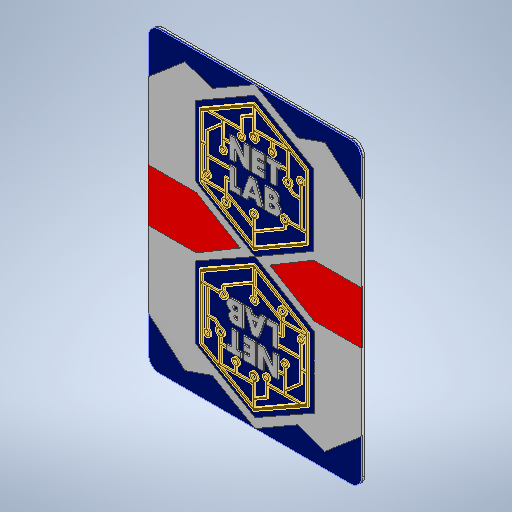
# Autodesk Inventor part: 3ofpython
Saved by Autodesk Inventor 2025 (Build 290162010, 162A)
## iProperties
Created: 2024-07-12
Part Number: 3ofpython
Material: Generic
Document SubType Name: Modeling
Designer: joshu
Density: 1 g/cm^3
Appearance: Default
Author: joshu
Autodesk Inventor part; units mm, degrees
(part 1 of 2)
ref_plane "YZ Plane" through (0, 0, 0) normal (1, 0, 0) x (0, 1, 0)
ref_plane "XZ Plane" through (0, 0, 0) normal (0, 1, 0) x (-1, 0, 0)
ref_plane "XY Plane" through (0, 0, 0) normal (0, 0, 1) x (1, 0, 0)
sketch "Sketch1" plane through (0, 0, 0) normal (0, 0, 1) x (1, 0, 0)
  line L0 (0, 0) -> (63.5, 0)
  line L1 (63.5, 0) -> (63.5, 88.9)
  line L2 (63.5, 88.9) -> (0, 88.9)
  line L3 (0, 88.9) -> (0, 0)
  line L4 (31.75, 44.45) -> (49.3079, 54.587)
  line L5 (49.3079, 54.587) -> (49.3079, 75.7826)
  line L6 (49.3079, 75.7826) -> (31.6801, 86.0828)
  line L7 (31.6801, 86.0828) -> (13.967, 75.8563)
  line L8 (13.967, 75.8563) -> (13.967, 55.04)
  line L9 (13.967, 55.04) -> (31.75, 44.45)
  line L10 (15.5263, 74.956) -> (31.6754, 84.2796)
  line L11 (31.6754, 84.2796) -> (47.7487, 74.8877)
  line L12 (47.7487, 74.8877) -> (47.7487, 55.4872)
  line L13 (47.7487, 55.4872) -> (31.7622, 46.2575)
  line L14 (31.7622, 46.2575) -> (15.5263, 55.9263)
  line L15 (15.5263, 55.9263) -> (15.5263, 74.956)
  line L16 (47.1273, 56.0392) -> (31.9379, 47.2671)
  line L17 (31.3664, 47.317) -> (16.2977, 56.192)
  line L18 (41.8086, 77.4972) -> (32.0418, 77.4972)
  line L19 (42.0908, 76.9257) -> (42.0908, 70.0939)
  line L20 (41.5193, 72.1376) -> (39.6994, 72.1376)
  line L21 (39.6994, 72.1376) -> (39.6994, 71.5661)
  line L22 (39.6994, 71.5661) -> (41.5193, 71.5661)
  arc A0 (31.465, 76.5861) -> (32.0365, 76.5861) centre (31.7507, 75.3324) ccw
  arc A1 (36.8763, 75.3571) -> (37.4478, 75.3571) centre (37.162, 74.2504) ccw
  circle A2 centre (37.162, 74.2504) radius 0.4762
  circle A3 centre (31.7507, 75.3324) radius 0.6191
  line L23 (45.9318, 69.8545) -> (45.9318, 58.9507)
  line L24 (45.3603, 66.7769) -> (43.3841, 66.7769)
  line L25 (43.1915, 66.2054) -> (45.3603, 66.2054)
  circle A4 centre (41.805, 68.7917) radius 0.762
  line L26 (43.1915, 66.2054) -> (41.9826, 67.4703)
  line L27 (43.3841, 66.7769) -> (42.5287, 67.6719)
  arc A5 (45.9318, 69.8545) -> (45.3603, 69.8545) centre (45.646, 70.9598) ccw
  circle A6 centre (45.646, 70.9598) radius 0.5715
  line L28 (40.6132, 56.5528) -> (40.6132, 57.4113)
  circle A7 centre (40.899, 58.665) radius 0.7144
  line L29 (32.0418, 83.1688) -> (32.0418, 77.4972)
  line L30 (32.0365, 76.9257) -> (32.0365, 76.5861)
  line L31 (32.0365, 76.9257) -> (36.8763, 76.9257)
  line L32 (36.8763, 75.3571) -> (36.8763, 76.9257)
  line L33 (37.4478, 76.9257) -> (37.4478, 75.3571)
  line L34 (37.4478, 76.9257) -> (41.5193, 76.9257)
  line L35 (42.0908, 76.9257) -> (42.7928, 76.9257)
  line L36 (32.0365, 83.1719) -> (41.8086, 77.4972)
  line L37 (42.7928, 76.9257) -> (47.1273, 74.4086)
  line L38 (41.5193, 70.0939) -> (41.5193, 71.5661)
  line L39 (41.5193, 72.1376) -> (41.5193, 76.9257)
  arc A8 (41.5193, 70.0939) -> (41.9826, 67.4703) centre (41.805, 68.7917) ccw
  arc A9 (42.5287, 67.6719) -> (42.0908, 70.0939) centre (41.805, 68.7917) ccw
  line L40 (45.3603, 58.9507) -> (45.3603, 66.2054)
  line L41 (45.3603, 66.7769) -> (45.3603, 69.8545)
  line L42 (47.1273, 58.9507) -> (45.9318, 58.9507)
  line L43 (45.3603, 58.9507) -> (42.1527, 58.9507)
  line L44 (42.1475, 58.3804) -> (47.1273, 58.3804)
  line L45 (41.1819, 57.4161) -> (41.1819, 56.2658)
  arc A10 (42.1527, 58.9507) -> (40.6132, 57.4113) centre (40.899, 58.665) ccw
  arc A11 (41.1819, 57.4161) -> (42.1475, 58.3804) centre (40.899, 58.665) ccw
  line L46 (47.1273, 74.4086) -> (47.1273, 58.9507)
  line L47 (47.1273, 58.3804) -> (47.1273, 56.0392)
  line L48 (27.6974, 78.6822) -> (27.6974, 79.0777)
  line L49 (28.2689, 78.6822) -> (31.465, 80.528)
  line L50 (27.6974, 79.0777) -> (31.465, 81.2535)
  line L51 (31.465, 76.5861) -> (31.465, 80.528)
  line L52 (31.465, 81.2535) -> (31.465, 83.1596)
  line L53 (31.9379, 51.4601) -> (40.6132, 56.5528)
  line L54 (31.9379, 50.8392) -> (41.1819, 56.2658)
  line L55 (16.2977, 57.1448) -> (22.9994, 57.1448)
  line L56 (22.9994, 56.5733) -> (16.2977, 56.5733)
  line L57 (16.2977, 56.5733) -> (16.2977, 57.1448)
  line L58 (22.9994, 60.9472) -> (23.5709, 60.9472)
  line L59 (22.9994, 60.9472) -> (24.4329, 60.9472)
  line L60 (24.4329, 60.9472) -> (24.4329, 60.3757)
  line L61 (24.4329, 60.3757) -> (23.5709, 60.3757)
  line L62 (22.9994, 60.3757) -> (22.9994, 60.9472)
  line L63 (23.5709, 56.4373) -> (31.3664, 51.9861)
  line L64 (31.3664, 52.5972) -> (23.5709, 57.0484)
  arc A12 (31.9379, 54.3552) -> (31.3664, 54.3552) centre (31.6521, 55.5111) ccw
  circle A13 centre (31.6521, 55.5111) radius 0.6191
  arc A14 (22.9994, 55.5805) -> (23.5709, 55.5805) centre (23.2852, 54.3309) ccw
  circle A15 centre (23.2852, 54.3309) radius 0.7144
  line L65 (23.5709, 60.3757) -> (23.5709, 57.0484)
  line L66 (23.5709, 56.4373) -> (23.5709, 55.5805)
  line L67 (22.9994, 55.5805) -> (22.9994, 56.5733)
  line L68 (22.9994, 57.1448) -> (22.9994, 60.9472)
  line L69 (31.3664, 54.3552) -> (31.3664, 52.5972)
  line L70 (31.3664, 51.9861) -> (31.3664, 47.317)
  line L71 (31.9379, 47.2671) -> (31.9379, 50.8392)
  line L72 (31.9379, 51.4601) -> (31.9379, 54.3552)
  arc A16 (27.6974, 74.6924) -> (28.2689, 74.6924) centre (27.9831, 73.6844) ccw
  circle A17 centre (27.9831, 73.6844) radius 0.4763
  line L73 (18.5492, 75.7007) -> (27.6974, 75.7007)
  line L74 (22.769, 70.6818) -> (24.4329, 70.6818)
  line L75 (24.4329, 70.6818) -> (24.4329, 70.1103)
  line L76 (24.4329, 70.1103) -> (22.769, 70.1103)
  line L77 (22.769, 70.1103) -> (22.769, 70.2009)
  line L78 (16.2977, 66.7769) -> (17.4065, 66.7769)
  line L79 (17.978, 66.7769) -> (17.978, 66.2054)
  line L80 (17.4065, 66.2054) -> (16.2977, 66.2054)
  line L81 (17.978, 63.9706) -> (24.4329, 63.9706)
  line L82 (24.4329, 63.9706) -> (24.4329, 63.3991)
  line L83 (24.4329, 63.3991) -> (17.978, 63.3991)
  line L84 (17.4065, 66.7769) -> (17.4065, 70.2549)
  line L85 (17.978, 70.0307) -> (17.978, 66.7769)
  line L86 (17.4065, 70.2549) -> (22.1975, 74.4365)
  line L87 (17.978, 70.0307) -> (22.1975, 73.7135)
  arc A18 (22.1975, 68.5281) -> (22.769, 68.5281) centre (22.4833, 67.4703) ccw
  circle A19 centre (22.4833, 67.4703) radius 0.5239
  line L88 (16.2977, 74.4004) -> (17.5596, 75.1292)
  line L89 (18.5492, 75.7007) -> (31.465, 83.1596)
  line L90 (27.6974, 75.1292) -> (22.769, 75.1292)
  line L91 (22.1975, 75.1292) -> (17.5596, 75.1292)
  line L92 (22.1975, 74.4365) -> (22.1975, 75.1292)
  line L93 (28.2689, 74.6924) -> (28.2689, 78.6822)
  line L94 (22.769, 75.1292) -> (22.769, 70.6818)
  line L95 (22.769, 70.1103) -> (22.769, 68.5281)
  line L96 (22.1975, 67.8875) -> (22.1975, 67.9094)
  line L97 (22.1975, 68.5281) -> (22.1975, 73.7135)
  line L98 (16.2977, 56.192) -> (16.2977, 66.2054)
  line L99 (16.2977, 66.7769) -> (16.2977, 74.4004)
  line L100 (17.978, 63.9706) -> (17.978, 66.2054)
  line L101 (27.6974, 78.6822) -> (27.6974, 75.7007)
  line L102 (27.6974, 75.1292) -> (27.6974, 74.6924)
  line L103 (24.4329, 66.1976) -> (26.1474, 66.1976)
  line L104 (26.1474, 66.1976) -> (26.1474, 69.7075)
  line L105 (26.1474, 72.4542) -> (24.4329, 72.4542)
  line L106 (24.4329, 72.4542) -> (24.4329, 66.1976)
  line L107 (28.7777, 72.4542) -> (30.4922, 72.4542)
  line L108 (30.4922, 72.4542) -> (30.4922, 66.1976)
  line L109 (30.4922, 66.1976) -> (28.7777, 66.1976)
  line L110 (28.7777, 68.9443) -> (28.7777, 72.4542)
  line L111 (28.7777, 66.1976) -> (26.1474, 69.7075)
  line L112 (26.1474, 72.4542) -> (28.7777, 68.9443)
  line L113 (31.2537, 72.4542) -> (32.9682, 72.4542)
  line L114 (32.9682, 66.1976) -> (31.2537, 66.1976)
  line L115 (31.2537, 66.1976) -> (31.2537, 72.4542)
  line L116 (31.2537, 72.4542) -> (34.8385, 72.4542)
  line L117 (34.8385, 72.4542) -> (34.8385, 70.7397)
  line L118 (34.8385, 70.7397) -> (32.9682, 70.7397)
  line L119 (31.2537, 70.7397) -> (31.2537, 72.4542)
  line L120 (32.9682, 70.0633) -> (34.8385, 70.0633)
  line L121 (34.8385, 70.0633) -> (34.8385, 68.5393)
  line L122 (34.8385, 68.5393) -> (32.9682, 68.5393)
  line L123 (31.2537, 68.5393) -> (31.2537, 70.0633)
  line L124 (31.2537, 66.1976) -> (34.8385, 66.1976)
  line L125 (34.8385, 66.1976) -> (34.8385, 67.9121)
  line L126 (34.8385, 67.9121) -> (32.9682, 67.9121)
  line L127 (31.2537, 67.9121) -> (31.2537, 66.1976)
  line L128 (32.9682, 70.7397) -> (32.9682, 70.0633)
  line L129 (32.9682, 68.5393) -> (32.9682, 67.9121)
  line L130 (39.6994, 72.4422) -> (35.4849, 72.4422)
  line L131 (35.4849, 72.4422) -> (35.4849, 70.9182)
  line L132 (39.6994, 70.9182) -> (39.6994, 72.4422)
  line L133 (38.4466, 70.9182) -> (38.4466, 66.1976)
  line L134 (38.4466, 66.1976) -> (36.7321, 66.1976)
  line L135 (36.7321, 66.1976) -> (36.7321, 70.9182)
  line L136 (36.7321, 70.9182) -> (36.8763, 70.9182)
  line L137 (35.4849, 70.9182) -> (36.7321, 70.9182)
  line L138 (38.4466, 70.9182) -> (39.6994, 70.9182)
  line L139 (24.4329, 64.6461) -> (26.1474, 64.6461)
  line L140 (26.1474, 64.6461) -> (26.1474, 59.9044)
  line L141 (26.1474, 58.3804) -> (24.4329, 58.3804)
  line L142 (24.4329, 58.3804) -> (24.4329, 64.6461)
  line L143 (24.4329, 58.3804) -> (27.8234, 58.3804)
  line L144 (27.8234, 58.3804) -> (27.8234, 59.9044)
  line L145 (27.8234, 59.9044) -> (26.1474, 59.9044)
  line L146 (24.4329, 59.9044) -> (24.4329, 58.3804)
  line L147 (28.1466, 58.3804) -> (29.8611, 58.3804)
  line L148 (29.8611, 58.3804) -> (30.3254, 59.5144)
  line L149 (30.3254, 59.5144) -> (32.2304, 59.5144)
  line L150 (30.3254, 64.6461) -> (32.2304, 64.6461)
  line L151 (28.1466, 58.3804) -> (30.3254, 64.6461)
  line L152 (32.728, 58.3804) -> (34.4425, 58.3804)
  line L153 (32.728, 58.3804) -> (32.2304, 59.5144)
  line L154 (34.4425, 58.3804) -> (32.2304, 64.6461)
  line L155 (30.6203, 60.8236) -> (31.9379, 60.8236)
  line L156 (31.9379, 60.8236) -> (31.2779, 62.4085)
  line L157 (31.2779, 62.4085) -> (30.6203, 60.8236)
  line L158 (34.9216, 58.3804) -> (34.9216, 64.6461)
  line L159 (34.9216, 64.6461) -> (37.8691, 64.6461)
  line L160 (34.9216, 58.3804) -> (37.8691, 58.3804)
  line L161 (36.5599, 59.8143) -> (36.5599, 60.939)
  line L162 (36.5599, 62.1736) -> (36.5599, 63.1944)
  line L163 (36.5599, 63.1944) -> (37.2133, 63.1944)
  line L164 (36.5599, 62.1736) -> (37.2133, 62.1736)
  arc A20 (37.2133, 62.1736) -> (37.2133, 63.1944) centre (37.055, 62.684) ccw
  line L165 (36.5599, 60.939) -> (37.4519, 60.939)
  line L166 (36.5599, 59.8143) -> (37.4396, 59.8143)
  arc A21 (37.4396, 59.8143) -> (37.4519, 60.939) centre (37.3959, 60.3772) ccw
  arc A22 (38.5631, 61.7817) -> (37.8691, 64.6461) centre (37.5266, 63.0469) ccw
  arc A23 (37.8691, 58.3804) -> (38.5631, 61.7817) centre (37.9604, 60.1332) ccw
  arc A24 (17.4065, 59.8724) -> (17.978, 59.8724) centre (17.6923, 58.815) ccw
  circle A25 centre (17.6923, 58.815) radius 0.5239
  line L167 (17.4065, 66.2054) -> (17.4065, 59.8724)
  line L168 (17.978, 59.8724) -> (17.978, 63.3991)
  line L169 (32.0418, 83.1688) -> (41.8086, 77.4972)
  line L170 (32.0418, 77.4972) -> (41.8086, 77.4972)
  line L171 (32.0418, 77.4972) -> (32.0418, 83.1688)
  line L172 (0, 44.45) -> (63.5, 44.45) construction
  line L173 (31.75, 88.9) -> (31.75, 0) construction
  line L174 (0, 52.2573) -> (14.2102, 52.2573)
  line L175 (14.2102, 52.2573) -> (27.3204, 44.45)
  line L176 (0, 36.6427) -> (14.2102, 36.6427)
  line L177 (14.2102, 36.6427) -> (27.3204, 44.45)
  line L178 (63.5, 52.2573) -> (49.2898, 52.2573)
  line L179 (49.2898, 52.2573) -> (36.1796, 44.45)
  line L180 (49.2898, 36.6427) -> (36.1796, 44.45)
  line L181 (63.5, 36.6427) -> (49.2898, 36.6427)
  line L182 (0, 75.0796) -> (10.8905, 84.3747)
  line L183 (10.8905, 84.3747) -> (18.9583, 81.5148)
  line L184 (18.9583, 81.5148) -> (31.75, 88.9)
  line L185 (63.5, 75.0796) -> (52.6095, 84.3747)
  line L186 (52.6095, 84.3747) -> (44.5417, 81.5148)
  line L187 (44.5417, 81.5148) -> (31.75, 88.9)
  line L188 (46.0393, 22.6946) -> (47.1481, 22.6946)
  line L189 (45.4678, 22.1231) -> (45.4678, 22.6946)
  line L190 (45.4678, 24.9294) -> (45.4678, 22.6946)
  line L191 (47.1481, 22.1231) -> (46.0393, 22.1231)
  line L192 (47.1481, 32.3267) -> (47.1481, 31.7552)
  line L193 (47.1481, 32.708) -> (47.1481, 22.6946)
  line L194 (47.1481, 31.7552) -> (40.4464, 31.7552)
  line L195 (40.4464, 32.3267) -> (47.1481, 32.3267)
  line L196 (45.4678, 29.0276) -> (45.4678, 25.5009)
  line L197 (46.0393, 22.6946) -> (46.0393, 29.0276)
  circle A26 centre (45.7535, 30.085) radius 0.5239
  arc A27 (46.0393, 29.0276) -> (45.4678, 29.0276) centre (45.7535, 30.085) ccw
  line L198 (20.6531, 11.9743) -> (16.3185, 14.4914)
  line L199 (21.355, 11.9743) -> (20.6531, 11.9743)
  line L200 (21.9265, 16.7624) -> (21.9265, 11.9743)
  line L201 (21.355, 11.9743) -> (21.355, 18.8061)
  line L202 (21.9265, 16.7624) -> (23.7464, 16.7624)
  line L203 (23.7464, 17.3339) -> (21.9265, 17.3339)
  line L204 (25.998, 11.9743) -> (21.9265, 11.9743)
  line L205 (26.5695, 13.5429) -> (26.5695, 11.9743)
  circle A28 centre (21.6408, 20.1083) radius 0.762
  circle A29 centre (26.2838, 14.6496) radius 0.4762
  arc A30 (26.5695, 13.5429) -> (25.998, 13.5429) centre (26.2838, 14.6496) ccw
  line L206 (31.4093, 11.9743) -> (26.5695, 11.9743)
  arc A31 (31.9808, 12.3139) -> (31.4093, 12.3139) centre (31.6951, 13.5676) ccw
  line L207 (25.998, 11.9743) -> (25.998, 13.5429)
  line L208 (45.4678, 24.9294) -> (39.013, 24.9294)
  line L209 (39.013, 25.5009) -> (45.4678, 25.5009)
  line L210 (39.013, 24.9294) -> (39.013, 25.5009)
  circle A32 centre (40.1606, 34.5691) radius 0.7144
  arc A33 (40.4464, 33.3195) -> (39.8749, 33.3195) centre (40.1606, 34.5691) ccw
  line L211 (39.8749, 32.4627) -> (39.8749, 33.3195)
  line L212 (40.4464, 33.3195) -> (40.4464, 32.3267)
  line L213 (39.013, 27.9528) -> (39.013, 28.5243)
  line L214 (39.8749, 28.5243) -> (39.8749, 31.8516)
  line L215 (39.013, 28.5243) -> (39.8749, 28.5243)
  line L216 (40.4464, 31.7552) -> (40.4464, 27.9528)
  line L217 (40.4464, 28.5243) -> (40.4464, 27.9528)
  line L218 (40.4464, 27.9528) -> (39.8749, 27.9528)
  line L219 (40.4464, 27.9528) -> (39.013, 27.9528)
  line L220 (33.5847, 30.5196) -> (33.1204, 29.3856)
  line L221 (35.6224, 28.9956) -> (37.2985, 28.9956)
  line L222 (35.2992, 30.5196) -> (33.5847, 30.5196)
  line L223 (39.013, 28.9956) -> (39.013, 30.5196)
  line L224 (35.2992, 30.5196) -> (33.1204, 24.2539)
  line L225 (46.0393, 18.6451) -> (41.2483, 14.4635)
  line L226 (45.4678, 18.8693) -> (41.2483, 15.1865)
  line L227 (40.6768, 18.7897) -> (40.6768, 20.3719)
  line L228 (41.2483, 21.0125) -> (41.2483, 20.9906)
  line L229 (41.2483, 20.3719) -> (41.2483, 15.1865)
  line L230 (40.6768, 13.7708) -> (40.6768, 18.2182)
  line L231 (41.2483, 14.4635) -> (41.2483, 13.7708)
  line L232 (41.2483, 13.7708) -> (45.8862, 13.7708)
  line L233 (47.1481, 22.1231) -> (47.1481, 14.4996)
  line L234 (47.1481, 14.4996) -> (45.8862, 13.7708)
  circle A34 centre (40.9626, 21.4297) radius 0.5239
  line L235 (32.8255, 28.0764) -> (31.5079, 28.0764)
  line L236 (32.1679, 26.4915) -> (32.8255, 28.0764)
  line L237 (31.5079, 28.0764) -> (32.1679, 26.4915)
  line L238 (33.1204, 29.3856) -> (31.2154, 29.3856)
  line L239 (35.6224, 30.5196) -> (35.6224, 28.9956)
  line L240 (37.2985, 24.2539) -> (37.2985, 28.9956)
  line L241 (37.2985, 30.5196) -> (39.013, 30.5196)
  line L242 (39.013, 30.5196) -> (39.013, 24.2539)
  line L243 (39.013, 30.5196) -> (35.6224, 30.5196)
  line L244 (39.013, 24.2539) -> (37.2985, 24.2539)
  line L245 (33.1204, 24.2539) -> (31.2154, 24.2539)
  line L246 (30.7178, 30.5196) -> (31.2154, 29.3856)
  line L247 (37.2985, 16.4458) -> (39.013, 16.4458)
  line L248 (40.6768, 18.2182) -> (39.013, 18.2182)
  line L249 (39.013, 18.7897) -> (40.6768, 18.7897)
  line L250 (40.6768, 18.7897) -> (40.6768, 18.6991)
  line L251 (39.013, 18.2182) -> (39.013, 18.7897)
  line L252 (46.0393, 22.1231) -> (46.0393, 18.6451)
  line L253 (45.4678, 18.8693) -> (45.4678, 22.1231)
  arc A35 (41.2483, 20.3719) -> (40.6768, 20.3719) centre (40.9626, 21.4297) ccw
  line L254 (39.013, 16.4458) -> (39.013, 22.7024)
  line L255 (39.013, 22.7024) -> (37.2985, 22.7024)
  line L256 (32.9536, 22.7024) -> (34.6681, 22.7024)
  line L257 (30.4777, 22.7024) -> (32.1922, 22.7024)
  line L258 (30.4777, 18.8367) -> (28.6073, 18.8367)
  line L259 (32.1922, 22.7024) -> (28.6073, 22.7024)
  line L260 (28.6073, 22.7024) -> (28.6073, 20.9879)
  line L261 (28.6073, 20.9879) -> (30.4777, 20.9879)
  line L262 (32.1922, 20.9879) -> (32.1922, 22.7024)
  line L263 (30.4777, 20.3607) -> (30.4777, 20.9879)
  line L264 (28.6073, 20.3607) -> (30.4777, 20.3607)
  line L265 (28.6073, 18.8367) -> (28.6073, 20.3607)
  line L266 (32.1922, 20.3607) -> (32.1922, 18.8367)
  line L267 (30.4777, 18.1603) -> (30.4777, 18.8367)
  line L268 (26.8859, 25.7056) -> (26.2325, 25.7056)
  line L269 (26.8859, 29.0857) -> (26.0062, 29.0857)
  line L270 (26.8859, 27.961) -> (25.9939, 27.961)
  line L271 (28.5242, 30.5196) -> (25.5767, 30.5196)
  line L272 (32.0794, 36.9139) -> (32.0794, 41.583)
  line L273 (31.5079, 41.6329) -> (31.5079, 38.0608)
  line L274 (26.8859, 26.7264) -> (26.8859, 25.7056)
  line L275 (28.5242, 24.2539) -> (25.5767, 24.2539)
  line L276 (29.0033, 30.5196) -> (31.2154, 24.2539)
  line L277 (30.7178, 30.5196) -> (29.0033, 30.5196)
  line L278 (26.8859, 26.7264) -> (26.2325, 26.7264)
  line L279 (28.5242, 30.5196) -> (28.5242, 24.2539)
  arc A36 (26.2325, 26.7264) -> (26.2325, 25.7056) centre (26.3908, 26.216) ccw
  line L280 (26.8859, 29.0857) -> (26.8859, 27.961)
  arc A37 (26.0062, 29.0857) -> (25.9939, 27.961) centre (26.0499, 28.5228) ccw
  arc A38 (24.8827, 27.1183) -> (25.5767, 24.2539) centre (25.9192, 25.8531) ccw
  arc A39 (25.5767, 30.5196) -> (24.8827, 27.1183) centre (25.4854, 28.7668) ccw
  line L281 (23.7464, 16.7624) -> (23.7464, 17.3339)
  line L282 (24.9992, 22.7024) -> (26.7137, 22.7024)
  line L283 (27.961, 17.9818) -> (26.7137, 17.9818)
  line L284 (26.7137, 22.7024) -> (26.7137, 17.9818)
  line L285 (26.7137, 17.9818) -> (26.5695, 17.9818)
  line L286 (24.9992, 17.9818) -> (24.9992, 22.7024)
  line L287 (24.9992, 17.9818) -> (23.7464, 17.9818)
  line L288 (27.961, 16.4578) -> (27.961, 17.9818)
  line L289 (23.7464, 16.4578) -> (27.961, 16.4578)
  line L290 (23.7464, 17.9818) -> (23.7464, 16.4578)
  line L291 (31.75, 44.45) -> (14.1379, 34.5158)
  line L292 (15.6972, 33.6051) -> (31.7276, 42.6471)
  line L293 (16.3185, 32.8608) -> (31.5079, 41.6329)
  line L294 (31.5079, 37.4399) -> (22.8326, 32.3472)
  line L295 (31.5079, 38.0608) -> (22.2639, 32.6342)
  line L296 (31.5079, 37.4399) -> (31.5079, 34.5448)
  line L297 (35.7484, 10.2178) -> (35.7484, 9.8223)
  line L298 (35.1769, 10.2178) -> (31.9808, 8.372)
  line L299 (35.7484, 9.8223) -> (31.9808, 7.6465)
  line L300 (31.9808, 12.3139) -> (31.9808, 8.372)
  line L301 (31.9808, 7.6465) -> (31.9808, 5.7404)
  circle A40 centre (35.4627, 15.2156) radius 0.4763
  arc A41 (35.7484, 14.2076) -> (35.1769, 14.2076) centre (35.4627, 15.2156) ccw
  line L302 (35.7484, 13.7708) -> (35.7484, 14.2076)
  line L303 (35.7484, 13.7708) -> (40.6768, 13.7708)
  line L304 (44.8966, 13.1993) -> (35.7484, 13.1993)
  line L305 (35.1769, 14.2076) -> (35.1769, 10.2178)
  line L306 (35.7484, 10.2178) -> (35.7484, 13.1993)
  line L307 (44.8966, 13.1993) -> (31.9808, 5.7404)
  line L308 (31.4093, 11.9743) -> (31.4093, 12.3139)
  line L309 (47.9195, 13.7706) -> (31.7623, 4.657)
  circle A42 centre (31.6951, 13.5676) radius 0.6191
  line L310 (31.7499, 2.8598) -> (49.4788, 12.8599)
  line L311 (47.9195, 32.9751) -> (47.9195, 13.7706)
  line L312 (49.4788, 12.8599) -> (49.4788, 33.86)
  circle A43 centre (31.7937, 33.3889) radius 0.6191
  line L313 (32.0794, 41.583) -> (47.1481, 32.708)
  line L314 (49.4788, 33.86) -> (31.75, 44.45)
  line L315 (31.7276, 42.6471) -> (47.9195, 32.9751)
  line L316 (32.0794, 36.3028) -> (39.8749, 31.8516)
  line L317 (39.8749, 32.4627) -> (32.0794, 36.9139)
  line L318 (32.0794, 34.5448) -> (32.0794, 36.3028)
  arc A44 (31.5079, 34.5448) -> (32.0794, 34.5448) centre (31.7937, 33.3889) ccw
  circle A45 centre (17.7998, 17.9402) radius 0.5715
  line L319 (18.0855, 22.1231) -> (20.0617, 22.1231)
  line L320 (20.2543, 22.6946) -> (18.0855, 22.6946)
  line L321 (22.8326, 32.3472) -> (22.8326, 31.4887)
  circle A46 centre (22.5468, 30.235) radius 0.7144
  line L322 (21.2984, 30.5196) -> (16.3185, 30.5196)
  line L323 (22.2639, 31.4839) -> (22.2639, 32.6342)
  arc A47 (21.2931, 29.9493) -> (22.8326, 31.4887) centre (22.5468, 30.235) ccw
  arc A48 (22.2639, 31.4839) -> (21.2984, 30.5196) centre (22.5468, 30.235) ccw
  line L324 (16.3185, 30.5196) -> (16.3185, 32.8608)
  line L325 (14.1379, 34.5158) -> (14.1379, 13.1174)
  line L326 (15.6972, 14.0137) -> (15.6972, 33.6051)
  line L327 (17.514, 19.0455) -> (17.514, 29.9493)
  line L328 (20.2543, 22.6946) -> (21.4633, 21.4297)
  line L329 (20.0617, 22.1231) -> (20.9171, 21.2281)
  arc A49 (17.514, 19.0455) -> (18.0855, 19.0455) centre (17.7998, 17.9402) ccw
  line L330 (21.9265, 18.8061) -> (21.9265, 17.3339)
  arc A50 (20.9171, 21.2281) -> (21.355, 18.8061) centre (21.6408, 20.1083) ccw
  line L331 (18.0855, 22.1231) -> (18.0855, 19.0455)
  line L332 (16.3185, 14.4914) -> (16.3185, 29.9493)
  line L333 (16.3185, 29.9493) -> (17.514, 29.9493)
  line L334 (18.0855, 29.9493) -> (18.0855, 22.6946)
  line L335 (18.0855, 29.9493) -> (21.2931, 29.9493)
  arc A51 (21.9265, 18.8061) -> (21.4633, 21.4297) centre (21.6408, 20.1083) ccw
  line L336 (14.1379, 13.1174) -> (31.7499, 2.8598)
  line L337 (31.7623, 4.657) -> (15.6972, 14.0137)
  line L338 (21.6372, 11.4028) -> (31.404, 11.4028)
  line L339 (31.404, 11.4028) -> (31.404, 5.7312)
  line L340 (31.404, 5.7312) -> (21.6372, 11.4028)
  line L341 (37.2985, 22.7024) -> (37.2985, 19.1925)
  line L342 (34.6681, 16.4458) -> (32.9536, 16.4458)
  line L343 (32.9536, 16.4458) -> (32.9536, 22.7024)
  line L344 (34.6681, 22.7024) -> (37.2985, 19.1925)
  line L345 (28.6073, 18.1603) -> (30.4777, 18.1603)
  line L346 (32.1922, 16.4458) -> (28.6073, 16.4458)
  line L347 (28.6073, 16.4458) -> (28.6073, 18.1603)
  line L348 (32.1922, 22.7024) -> (32.1922, 16.4458)
  line L349 (32.1922, 16.4458) -> (30.4777, 16.4458)
  line L350 (34.6681, 19.9557) -> (34.6681, 16.4458)
  line L351 (37.2985, 16.4458) -> (34.6681, 19.9557)
  line L352 (32.1922, 18.1603) -> (32.1922, 16.4458)
  line L353 (0, 13.8204) -> (10.8905, 4.5253)
  line L354 (10.8905, 4.5253) -> (18.9583, 7.3852)
  line L355 (18.9583, 7.3852) -> (31.75, 0)
  line L356 (63.5, 13.8204) -> (52.6095, 4.5253)
  line L357 (52.6095, 4.5253) -> (44.5417, 7.3852)
  line L358 (44.5417, 7.3852) -> (31.75, 0)
  point P0 (31.9379, 47.317)
  point P1 (31.7229, 65.2666)
  point P2 (31.7229, 23.6334)
  point P3 (31.7229, 23.6334)
  point P4 (31.9379, 5.6837)
  point P5 (63.5, 75.0796)
  dimension "d0" = 63.5
  dimension "d1" = 88.9
  dimension "d43" = 44.45
  dimension "d99" = 120
  constraints: 718 end point, 170 parallel, 64 point on circle, 50 centre point, 42 perpendicular, 36 horizontal, 21 point on line, 20 coincident, 19 symmetric about line, 7 collinear, 5 midpoint, 4 vertical, 17 other
  measures "d0" distance of L2.end L1.end
  measures "d1" distance of L1.end L0.end
  measures "d43" distance between parallel lines of L172 L2
  measures "d99" angle of L357 L356
extrude "Extrusion1" add sketch "Sketch1" along normal blind 0.4 contours L3 L353 L354 L355 L0 | L358 L357 L356 L1 L0 | L3 L2 L184 L183 L182 | L185 L186 L187 L2 L1 | L9 L8 L7 L6 L5 L4 | L314 L312 L310 L336 L325 L291 | L10 L11 L12 L13 L14 L15 | L16 L71 L54 L45 A11 L44 L47 | L17 L98 L56 L67 A14 L66 L63 L70 | L18 L29 L36 | L35 L37 L46 L42 L23 A5 L41 L24 L27 A9 L19 | L20 L132 L130 L131 L137 L135 L134 L133 L138 L22 L38 A8 L26 L25 L40 L43 A10 L28 L53 L72 A12 L69 L64 L65 L61 L142 L141 L143 L144 L145 L140 L139 L81 L100 L79 L85 L87 L97 A18 L95 L76 L106 L103 L104 L111 L109 L108 L107 L110 L112 L105 L74 L94 L90 L102 A16 L93 L49 L51 A0 L30 L31 L32 A1 L33 L34 L39 | L21 L132 L138 L133 L134 L135 L137 L131 L130 | L106 L105 L112 L110 L107 L108 L109 L111 L104 L103 L75 | L60 L142 L82 L139 L140 L145 L144 L143 L141 | L59 L58 L62 L68 L55 L98 L80 L167 A24 L168 L83 L142 | A2 | A3 | A4 | A6 | A7 | L101 L73 L89 L52 L50 L48 | A13 | A15 | A17 | L99 L88 L91 L92 L86 L84 L78 | A19 | L113 L116 L117 L118 L128 L120 L121 L122 L129 L126 L125 L124 L114 L115 | L151 L150 L154 L152 L153 L149 L148 L147 | L157 L156 L155 | L158 L159 A22 A23 L160 | L161 L165 A21 L166 | L162 L163 A20 L164 | A25 | L197 A27 L196 L209 L242 L219 L218 L216 L194 L193 L188 | L210 L242 L244 L240 L221 L239 L243 L241 L223 L213 | L208 L190 L189 L253 L226 L229 A35 L227 L249 L254 L255 L341 L344 L256 L343 L342 L350 L351 L247 L248 L230 L303 L302 A41 L305 L298 L300 A31 L308 L206 L205 A30 L207 L204 L200 L202 L290 L289 L288 L283 L284 L282 L286 L287 L203 L330 A51 L328 L320 L334 L335 A47 L321 L294 L296 A44 L318 L316 L214 L215 L242 L223 L241 L243 L239 L221 L240 L244 | L251 L254 L247 L351 L350 L342 L343 L256 L344 L341 L255 | L290 L287 L286 L282 L284 L283 L288 L289 L281 | L233 L234 L232 L231 L225 L252 L191 | L193 L195 L212 A33 L211 L317 L272 L313 | A26 | L198 L332 L333 L327 A49 L331 L319 L329 A50 L201 L199 | A28 | A29 | A32 | L222 L224 L245 L276 L277 L246 L238 L220 | A34 | L236 L237 L235 | L257 L262 L348 L266 L346 L347 L345 L267 L258 L265 L264 L263 L261 L260 L259 | L268 A36 L278 L274 | L280 L270 A37 L269 | L279 L275 A38 A39 L271 | L273 L295 L323 A48 L322 L324 L293 | L292 L315 L311 L309 L337 L326 | L306 L304 L307 L301 L299 L297 | A40 | A42 | A43 | A45 | A46 | L338 L339 L340
extrude "Extrusion12" add sketch "Sketch1" along normal blind 0.4 separate body contours L3 L174 L175 L177 L176 | L181 L180 L179 L178 L1
extrude "Extrusion13" add sketch "Sketch1" along normal blind 0.4 separate body contours L355 L354 L353 L3 L176 L177 L175 L174 L182 L183 L184 L187 L186 L185 L1 L178 L179 L180 L181 L356 L357 L358
extrude "Extrusion14" add sketch "Sketch1" against normal blind 0.4 contours L21 L132 L138 L133 L134 L135 L137 L131 L130 | L106 L105 L112 L110 L107 L108 L109 L111 L104 L103 L75 | L60 L142 L82 L139 L140 L145 L144 L143 L141 | L113 L116 L117 L118 L128 L120 L121 L122 L129 L126 L125 L124 L114 L115 | L151 L150 L154 L152 L153 L149 L148 L147 | L158 L159 A22 A23 L160 | L210 L242 L244 L240 L221 L239 L243 L241 L223 L213 | L251 L254 L247 L351 L350 L342 L343 L256 L344 L341 L255 | L290 L287 L286 L282 L284 L283 L288 L289 L281 | L222 L224 L245 L276 L277 L246 L238 L220 | L257 L262 L348 L266 L346 L347 L345 L267 L258 L265 L264 L263 L261 L260 L259 | L279 L275 A38 A39 L271 bodies 3
extrude "Extrusion15" add sketch "Sketch1" against normal blind 0.4 separate body contours L10 L11 L12 L13 L14 L15 | L292 L315 L311 L309 L337 L326
pattern_linear "Rectangular Pattern1" count 2 spacing 0.8 along (0, 0, 1) of "Extrusion15" bodies 4
pattern_linear "Rectangular Pattern2" count 2 spacing 0.8 along (0, 0, 1) of "Extrusion14" bodies 3
extrude "Extrusion16" cut sketch "Sketch1" against normal blind 0.4 contours L9 L8 L7 L6 L5 L4 | L314 L312 L310 L336 L325 L291 | L10 L11 L12 L13 L14 L15 | L16 L71 L54 L45 A11 L44 L47 | L17 L98 L56 L67 A14 L66 L63 L70 | L18 L29 L36 | L35 L37 L46 L42 L23 A5 L41 L24 L27 A9 L19 | L20 L132 L130 L131 L137 L135 L134 L133 L138 L22 L38 A8 L26 L25 L40 L43 A10 L28 L53 L72 A12 L69 L64 L65 L61 L142 L141 L143 L144 L145 L140 L139 L81 L100 L79 L85 L87 L97 A18 L95 L76 L106 L103 L104 L111 L109 L108 L107 L110 L112 L105 L74 L94 L90 L102 A16 L93 L49 L51 A0 L30 L31 L32 A1 L33 L34 L39 | L21 L132 L138 L133 L134 L135 L137 L131 L130 | L106 L105 L112 L110 L107 L108 L109 L111 L104 L103 L75 | L60 L142 L82 L139 L140 L145 L144 L143 L141 | L59 L58 L62 L68 L55 L98 L80 L167 A24 L168 L83 L142 | A2 | A3 | A4 | A6 | A7 | L101 L73 L89 L52 L50 L48 | A13 | A15 | A17 | L99 L88 L91 L92 L86 L84 L78 | A19 | L113 L116 L117 L118 L128 L120 L121 L122 L129 L126 L125 L124 L114 L115 | L151 L150 L154 L152 L153 L149 L148 L147 | L157 L156 L155 | L158 L159 A22 A23 L160 | L161 L165 A21 L166 | L162 L163 A20 L164 | A25 | L197 A27 L196 L209 L242 L219 L218 L216 L194 L193 L188 | L210 L242 L244 L240 L221 L239 L243 L241 L223 L213 | L208 L190 L189 L253 L226 L229 A35 L227 L249 L254 L255 L341 L344 L256 L343 L342 L350 L351 L247 L248 L230 L303 L302 A41 L305 L298 L300 A31 L308 L206 L205 A30 L207 L204 L200 L202 L290 L289 L288 L283 L284 L282 L286 L287 L203 L330 A51 L328 L320 L334 L335 A47 L321 L294 L296 A44 L318 L316 L214 L215 L242 L223 L241 L243 L239 L221 L240 L244 | L251 L254 L247 L351 L350 L342 L343 L256 L344 L341 L255 | L290 L287 L286 L282 L284 L283 L288 L289 L281 | L233 L234 L232 L231 L225 L252 L191 | L193 L195 L212 A33 L211 L317 L272 L313 | A26 | L198 L332 L333 L327 A49 L331 L319 L329 A50 L201 L199 | A28 | A29 | A32 | L222 L224 L245 L276 L277 L246 L238 L220 | A34 | L236 L237 L235 | L257 L262 L348 L266 L346 L347 L345 L267 L258 L265 L264 L263 L261 L260 L259 | L268 A36 L278 L274 | L280 L270 A37 L269 | L279 L275 A38 A39 L271 | L273 L295 L323 A48 L322 L324 L293 | L292 L315 L311 L309 L337 L326 | L306 L304 L307 L301 L299 L297 | A40 | A42 | A43 | A45 | A46 | L338 L339 L340 bodies 3
extrude "Extrusion17" cut sketch "Sketch1" against normal blind 25.4 contours L9 L8 L7 L6 L5 L4 | L314 L312 L310 L336 L325 L291 | L10 L11 L12 L13 L14 L15 | L16 L71 L54 L45 A11 L44 L47 | L17 L98 L56 L67 A14 L66 L63 L70 | L18 L29 L36 | L35 L37 L46 L42 L23 A5 L41 L24 L27 A9 L19 | L20 L132 L130 L131 L137 L135 L134 L133 L138 L22 L38 A8 L26 L25 L40 L43 A10 L28 L53 L72 A12 L69 L64 L65 L61 L142 L141 L143 L144 L145 L140 L139 L81 L100 L79 L85 L87 L97 A18 L95 L76 L106 L103 L104 L111 L109 L108 L107 L110 L112 L105 L74 L94 L90 L102 A16 L93 L49 L51 A0 L30 L31 L32 A1 L33 L34 L39 | L21 L132 L138 L133 L134 L135 L137 L131 L130 | L106 L105 L112 L110 L107 L108 L109 L111 L104 L103 L75 | L60 L142 L82 L139 L140 L145 L144 L143 L141 | L59 L58 L62 L68 L55 L98 L80 L167 A24 L168 L83 L142 | A2 | A3 | A4 | A6 | A7 | L101 L73 L89 L52 L50 L48 | A13 | A15 | A17 | L99 L88 L91 L92 L86 L84 L78 | A19 | L113 L116 L117 L118 L128 L120 L121 L122 L129 L126 L125 L124 L114 L115 | L151 L150 L154 L152 L153 L149 L148 L147 | L157 L156 L155 | L158 L159 A22 A23 L160 | L161 L165 A21 L166 | L162 L163 A20 L164 | A25 | L197 A27 L196 L209 L242 L219 L218 L216 L194 L193 L188 | L210 L242 L244 L240 L221 L239 L243 L241 L223 L213 | L208 L190 L189 L253 L226 L229 A35 L227 L249 L254 L255 L341 L344 L256 L343 L342 L350 L351 L247 L248 L230 L303 L302 A41 L305 L298 L300 A31 L308 L206 L205 A30 L207 L204 L200 L202 L290 L289 L288 L283 L284 L282 L286 L287 L203 L330 A51 L328 L320 L334 L335 A47 L321 L294 L296 A44 L318 L316 L214 L215 L242 L223 L241 L243 L239 L221 L240 L244 | L251 L254 L247 L351 L350 L342 L343 L256 L344 L341 L255 | L290 L287 L286 L282 L284 L283 L288 L289 L281 | L233 L234 L232 L231 L225 L252 L191 | L193 L195 L212 A33 L211 L317 L272 L313 | A26 | L198 L332 L333 L327 A49 L331 L319 L329 A50 L201 L199 | A28 | A29 | A32 | L222 L224 L245 L276 L277 L246 L238 L220 | A34 | L236 L237 L235 | L257 L262 L348 L266 L346 L347 L345 L267 L258 L265 L264 L263 L261 L260 L259 | L268 A36 L278 L274 | L280 L270 A37 L269 | L279 L275 A38 A39 L271 | L273 L295 L323 A48 L322 L324 L293 | L292 L315 L311 L309 L337 L326 | L306 L304 L307 L301 L299 L297 | A40 | A42 | A43 | A45 | A46 | L338 L339 L340 bodies 4
sketch "Sketch14" plane through (0, 0, 0) normal (0, 0, -1) x (-1, 0, 0)
  line L0 (-63.5, 75.0796) -> (-63.5, 88.9) projected
  line L1 (0, 0) -> (-63.5, 0)
  line L2 (-63.5, 0) -> (-63.5, 88.9)
  line L3 (-63.5, 88.9) -> (0, 88.9)
  line L4 (0, 88.9) -> (0, 0)
  line L5 (-62.5, 1) -> (-1, 1)
  line L6 (-1, 1) -> (-1, 87.9)
  line L7 (-1, 87.9) -> (-62.5, 87.9)
  line L8 (-62.5, 87.9) -> (-62.5, 1)
  dimension "d90" = 1
  constraints: 16 end point, 4 parallel, 2 perpendicular, 1 horizontal, 3 other
  measures "d90" distance between parallel lines of L1 L5
extrude "Extrusion18" add sketch "Sketch14" along normal blind 0.2 separate body contours L8 L7 L6 L5
sketch "Sketch16" plane through (0, 0, 0) normal (0, 0, -1) x (-1, 0, 0)
  line L0 (-1, 1) -> (-1, 87.9) projected
  line L1 (-1, 87.9) -> (-62.5, 87.9) projected
  line L2 (-62.5, 87.9) -> (-62.5, 1) projected
  line L3 (-62.5, 1) -> (-1, 1) projected
  line L4 (0, 88.9) -> (0, 75.0796) projected
  line L5 (-31.75, 0) -> (-63.5, 0) projected
  line L6 (0, 88.9) -> (-63.5, 88.9)
  line L7 (-63.5, 88.9) -> (-63.5, 0)
  line L8 (-63.5, 0) -> (0, 0)
  line L9 (0, 0) -> (0, 88.9)
  constraints: 8 end point, 2 parallel, 1 horizontal, 1 perpendicular
extrude "Extrusion19" add sketch "Sketch16" along normal blind 0.2 bodies 3
sketch "Sketch17" plane through (0, 0, -0.2) normal (0, 0, -1) x (-1, 0, 0)
  line L0 (-63.5, 88.9) -> (-63.5, 0)
  line L1 (-63.5, 0) -> (0, 0)
  line L2 (0, 0) -> (0, 88.9)
  line L3 (0, 88.9) -> (-63.5, 88.9)
  line L4 (-62.5, 1) -> (-62.5, 87.9) construction
  line L5 (-62.5, 44.45) -> (-1, 44.45) construction
  line L6 (-1, 87.9) -> (-1, 1) construction
  line L7 (-57.9556, 87.392) -> (-49.5403, 87.392) construction
  line L8 (-49.5403, 87.392) -> (-49.5403, 73.7102) construction
  line L9 (-49.5403, 73.7102) -> (-57.9556, 73.7102) construction
  line L10 (-57.9556, 73.7102) -> (-57.9556, 87.392) construction
  line L11 (-5.5444, 1.508) -> (-13.9597, 1.508) construction
  line L12 (-13.9597, 1.508) -> (-13.9597, 15.8789) construction
  line L13 (-13.9597, 15.8789) -> (-5.5444, 15.8789) construction
  line L14 (-5.5444, 15.8789) -> (-5.5444, 1.508) construction
  line L15 (-62.5, 87.9) -> (-1, 87.9) projected
  line L16 (-1, 1) -> (-62.5, 1) projected
  line L17 (-15.9555, 100.6878) -> (-15.9555, 101.8081)
  arc A0 (-15.758, 102.5167) -> (-15.9555, 101.8081) centre (-14.5235, 101.7908) ccw
  arc A1 (-14.8139, 103.0351) -> (-15.758, 102.5167) centre (-14.7944, 101.8807) ccw
  line L18 (-14.8139, 103.0351) -> (-12.5434, 103.0404)
  arc A2 (-12.5434, 103.0404) -> (-11.3034, 104.2101) centre (-12.4298, 104.1621) ccw
  line L19 (-11.3034, 104.2101) -> (-11.308, 106.1909)
  arc A3 (-11.308, 106.1909) -> (-11.7101, 106.9805) centre (-12.2888, 106.1886) ccw
  arc A4 (-11.7101, 106.9805) -> (-12.7195, 107.3451) centre (-13.0065, 104.9711) ccw
  arc A5 (-12.7195, 107.3451) -> (-14.3215, 107.3451) centre (-13.5205, 101.117) ccw
  arc A6 (-14.3215, 107.3451) -> (-15.3501, 106.9805) centre (-14.123, 105.152) ccw
  arc A7 (-15.3501, 106.9805) -> (-15.6604, 106.4938) centre (-14.9717, 106.397) ccw
  line L20 (-15.6604, 106.4938) -> (-15.6604, 105.3776)
  line L21 (-15.6604, 105.3776) -> (-13.4817, 105.3776)
  line L22 (-13.4817, 105.3776) -> (-13.4817, 105.0592)
  line L23 (-13.4817, 105.0592) -> (-16.5554, 105.0592)
  arc A8 (-16.5554, 105.0592) -> (-17.8802, 103.9116) centre (-16.4912, 103.6466) ccw
  arc A9 (-17.8802, 103.9116) -> (-17.7338, 101.4545) centre (-14.109, 102.9033) ccw
  arc A10 (-17.7338, 101.4545) -> (-16.815, 100.6878) centre (-16.5647, 101.9218) ccw
  line L24 (-16.815, 100.6878) -> (-15.9555, 100.6878)
  line L25 (-10.9984, 105.1392) -> (-10.9984, 104.019)
  arc A11 (-11.1959, 103.3104) -> (-10.9984, 104.019) centre (-12.4304, 104.0362) ccw
  arc A12 (-12.14, 102.792) -> (-11.1959, 103.3104) centre (-12.1595, 103.9464) ccw
  line L26 (-12.14, 102.792) -> (-14.4105, 102.7867)
  arc A13 (-14.4105, 102.7867) -> (-15.6506, 101.6169) centre (-14.5241, 101.6649) ccw
  line L27 (-15.6506, 101.6169) -> (-15.6459, 99.6361)
  arc A14 (-15.6459, 99.6361) -> (-15.2438, 98.8466) centre (-14.6652, 99.6384) ccw
  arc A15 (-15.2438, 98.8466) -> (-14.2344, 98.4819) centre (-13.9475, 100.8559) ccw
  arc A16 (-14.2344, 98.4819) -> (-12.6324, 98.4819) centre (-13.4334, 104.71) ccw
  arc A17 (-12.6324, 98.4819) -> (-11.6038, 98.8466) centre (-12.8309, 100.6751) ccw
  arc A18 (-11.6038, 98.8466) -> (-11.2936, 99.3332) centre (-11.9822, 99.43) ccw
  line L28 (-11.2936, 99.3332) -> (-11.2936, 100.4494)
  line L29 (-11.2936, 100.4494) -> (-13.4723, 100.4494)
  line L30 (-13.4723, 100.4494) -> (-13.4723, 100.7678)
  line L31 (-13.4723, 100.7678) -> (-10.3985, 100.7678)
  arc A19 (-10.3985, 100.7678) -> (-9.0738, 101.9154) centre (-10.4627, 102.1804) ccw
  arc A20 (-9.0738, 101.9154) -> (-9.2201, 104.3725) centre (-12.8449, 102.9238) ccw
  arc A21 (-9.2201, 104.3725) -> (-10.1389, 105.1392) centre (-10.3892, 103.9053) ccw
  line L32 (-10.1389, 105.1392) -> (-10.9984, 105.1392)
  circle A22 centre (-14.7136, 106.2998) radius 0.3922
  circle A23 centre (-12.2308, 99.4812) radius 0.4142
  line L33 (-35.0174, 65.9538) -> (-35.0174, 67.4278)
  arc A24 (-34.7576, 68.3601) -> (-35.0174, 67.4278) centre (-33.1333, 67.4051) ccw
  arc A25 (-33.5153, 69.0422) -> (-34.7576, 68.3601) centre (-33.4897, 67.5233) ccw
  line L34 (-33.5153, 69.0422) -> (-30.5278, 69.0492)
  arc A26 (-30.5278, 69.0492) -> (-28.8962, 70.5884) centre (-30.3784, 70.5252) ccw
  line L35 (-28.8962, 70.5884) -> (-28.9023, 73.1947)
  arc A27 (-28.9023, 73.1947) -> (-29.4314, 74.2336) centre (-30.1928, 73.1916) ccw
  arc A28 (-29.4314, 74.2336) -> (-30.7595, 74.7133) centre (-31.1371, 71.5897) ccw
  arc A29 (-30.7595, 74.7133) -> (-32.8674, 74.7133) centre (-31.8135, 66.5185) ccw
  arc A30 (-32.8674, 74.7133) -> (-34.2209, 74.2336) centre (-32.6063, 71.8276) ccw
  arc A31 (-34.2209, 74.2336) -> (-34.6291, 73.5932) centre (-33.7229, 73.4659) ccw
  line L36 (-34.6291, 73.5932) -> (-34.6291, 72.1245)
  line L37 (-34.6291, 72.1245) -> (-31.7624, 72.1245)
  line L38 (-31.7624, 72.1245) -> (-31.7624, 71.7056)
  line L39 (-31.7624, 71.7056) -> (-35.8068, 71.7056)
  arc A32 (-35.8068, 71.7056) -> (-37.5499, 70.1956) centre (-35.7223, 69.8469) ccw
  arc A33 (-37.5499, 70.1956) -> (-37.3573, 66.9625) centre (-32.5879, 68.8688) ccw
  arc A34 (-37.3573, 66.9625) -> (-36.1484, 65.9538) centre (-35.819, 67.5774) ccw
  line L40 (-36.1484, 65.9538) -> (-35.0174, 65.9538)
  arc A35 (-32.9846, 68.7154) -> (-34.6162, 67.1763) centre (-33.134, 67.2394) ccw
  line L41 (-31.75, 65.6401) -> (-31.75, 66.059)
  arc A36 (-32.7529, 63.0513) -> (-30.645, 63.0513) centre (-31.6989, 71.2461) ccw
  arc A37 (-34.6101, 64.57) -> (-34.081, 63.5311) centre (-33.3196, 64.573) ccw
  line L42 (-34.6162, 67.1763) -> (-34.6101, 64.57)
  arc A38 (-30.645, 63.0513) -> (-29.2915, 63.5311) centre (-30.9061, 65.937) ccw
  line L43 (-28.8833, 65.6401) -> (-31.75, 65.6401)
  arc A39 (-29.2915, 63.5311) -> (-28.8833, 64.1714) centre (-29.7895, 64.2988) ccw
  line L44 (-29.9971, 68.7224) -> (-32.9846, 68.7154)
  line L45 (-31.75, 66.059) -> (-27.7056, 66.059)
  arc A40 (-28.7548, 69.4045) -> (-28.495, 70.3368) centre (-30.3791, 70.3595) ccw
  arc A41 (-29.9971, 68.7224) -> (-28.7548, 69.4045) centre (-30.0227, 70.2413) ccw
  arc A42 (-34.081, 63.5311) -> (-32.7529, 63.0513) centre (-32.3753, 66.1749) ccw
  line L46 (-28.8833, 64.1714) -> (-28.8833, 65.6401)
  line L47 (-28.495, 71.8108) -> (-28.495, 70.3368)
  arc A43 (-27.7056, 66.059) -> (-25.9625, 67.569) centre (-27.7901, 67.9177) ccw
  arc A44 (-26.155, 70.8021) -> (-27.364, 71.8108) centre (-27.6934, 70.1872) ccw
  arc A45 (-25.9625, 67.569) -> (-26.155, 70.8021) centre (-30.9245, 68.8958) ccw
  line L48 (-27.364, 71.8108) -> (-28.495, 71.8108)
  circle A46 centre (-33.3833, 73.338) radius 0.5161
  circle A47 centre (-30.1164, 64.3662) radius 0.545
  line L49 (-35.0174, 41.508) -> (-35.0174, 42.982)
  arc A48 (-34.7576, 43.9143) -> (-35.0174, 42.982) centre (-33.1333, 42.9593) ccw
  arc A49 (-33.5153, 44.5964) -> (-34.7576, 43.9143) centre (-33.4897, 43.0775) ccw
  line L50 (-33.5153, 44.5964) -> (-30.5278, 44.6034)
  arc A50 (-30.5278, 44.6034) -> (-28.8962, 46.1426) centre (-30.3784, 46.0794) ccw
  line L51 (-28.8962, 46.1426) -> (-28.9023, 48.7488)
  arc A51 (-28.9023, 48.7488) -> (-29.4314, 49.7878) centre (-30.1928, 48.7458) ccw
  arc A52 (-29.4314, 49.7878) -> (-30.7595, 50.2675) centre (-31.1371, 47.1439) ccw
  arc A53 (-30.7595, 50.2675) -> (-32.8674, 50.2675) centre (-31.8135, 42.0727) ccw
  arc A54 (-32.8674, 50.2675) -> (-34.2209, 49.7878) centre (-32.6063, 47.3818) ccw
  arc A55 (-34.2209, 49.7878) -> (-34.6291, 49.1474) centre (-33.7229, 49.02) ccw
  line L52 (-34.6291, 49.1474) -> (-34.6291, 47.6787)
  line L53 (-34.6291, 47.6787) -> (-31.7624, 47.6787)
  line L54 (-31.7624, 47.6787) -> (-31.7624, 47.2598)
  line L55 (-31.7624, 47.2598) -> (-35.8068, 47.2598)
  arc A56 (-35.8068, 47.2598) -> (-37.5499, 45.7498) centre (-35.7223, 45.4011) ccw
  arc A57 (-37.5499, 45.7498) -> (-37.3573, 42.5167) centre (-32.5879, 44.423) ccw
  arc A58 (-37.3573, 42.5167) -> (-36.1484, 41.508) centre (-35.819, 43.1316) ccw
  line L56 (-36.1484, 41.508) -> (-35.0174, 41.508)
  arc A59 (-32.9846, 44.2696) -> (-34.6162, 42.7305) centre (-33.134, 42.7936) ccw
  line L57 (-31.75, 41.1943) -> (-31.75, 41.6132)
  arc A60 (-32.7529, 38.6055) -> (-30.645, 38.6055) centre (-31.6989, 46.8003) ccw
  arc A61 (-34.6101, 40.1242) -> (-34.081, 39.0853) centre (-33.3196, 40.1272) ccw
  line L58 (-34.6162, 42.7305) -> (-34.6101, 40.1242)
  arc A62 (-30.645, 38.6055) -> (-29.2915, 39.0853) centre (-30.9061, 41.4912) ccw
  line L59 (-28.8833, 41.1943) -> (-31.75, 41.1943)
  arc A63 (-29.2915, 39.0853) -> (-28.8833, 39.7256) centre (-29.7895, 39.853) ccw
  line L60 (-29.9971, 44.2766) -> (-32.9846, 44.2696)
  line L61 (-31.75, 41.6132) -> (-27.7056, 41.6132)
  arc A64 (-28.7548, 44.9587) -> (-28.495, 45.891) centre (-30.3791, 45.9137) ccw
  arc A65 (-29.9971, 44.2766) -> (-28.7548, 44.9587) centre (-30.0227, 45.7955) ccw
  arc A66 (-34.081, 39.0853) -> (-32.7529, 38.6055) centre (-32.3753, 41.7291) ccw
  line L62 (-28.8833, 39.7256) -> (-28.8833, 41.1943)
  line L63 (-28.495, 47.365) -> (-28.495, 45.891)
  arc A67 (-27.7056, 41.6132) -> (-25.9625, 43.1232) centre (-27.7901, 43.4719) ccw
  arc A68 (-26.155, 46.3563) -> (-27.364, 47.365) centre (-27.6934, 45.7414) ccw
  arc A69 (-25.9625, 43.1232) -> (-26.155, 46.3563) centre (-30.9245, 44.45) ccw
  line L64 (-27.364, 47.365) -> (-28.495, 47.365)
  circle A70 centre (-33.3833, 48.8922) radius 0.5161
  circle A71 centre (-30.1164, 39.9204) radius 0.545
  line L65 (-28.4826, 22.9429) -> (-28.4826, 21.4689)
  arc A72 (-28.7424, 20.5365) -> (-28.4826, 21.4689) centre (-30.3667, 21.4916) ccw
  arc A73 (-29.9847, 19.8544) -> (-28.7424, 20.5365) centre (-30.0103, 21.3734) ccw
  line L66 (-29.9847, 19.8544) -> (-32.9722, 19.8474)
  arc A74 (-32.9722, 19.8474) -> (-34.6038, 18.3083) centre (-33.1216, 18.3715) ccw
  line L67 (-34.6038, 18.3083) -> (-34.5977, 15.702)
  arc A75 (-34.5977, 15.702) -> (-34.0686, 14.6631) centre (-33.3072, 15.705) ccw
  arc A76 (-34.0686, 14.6631) -> (-32.7405, 14.1834) centre (-32.3629, 17.307) ccw
  arc A77 (-32.7405, 14.1834) -> (-30.6326, 14.1834) centre (-31.6865, 22.3782) ccw
  arc A78 (-30.6326, 14.1834) -> (-29.2791, 14.6631) centre (-30.8937, 17.0691) ccw
  arc A79 (-29.2791, 14.6631) -> (-28.8709, 15.3035) centre (-29.7771, 15.4308) ccw
  line L68 (-28.8709, 15.3035) -> (-28.8709, 16.7721)
  line L69 (-28.8709, 16.7721) -> (-31.7376, 16.7721)
  line L70 (-31.7376, 16.7721) -> (-31.7376, 17.1911)
  line L71 (-31.7376, 17.1911) -> (-27.6932, 17.1911)
  arc A80 (-27.6932, 17.1911) -> (-25.9501, 18.7011) centre (-27.7777, 19.0497) ccw
  arc A81 (-25.9501, 18.7011) -> (-26.1427, 21.9341) centre (-30.9121, 20.0279) ccw
  arc A82 (-26.1427, 21.9341) -> (-27.3516, 22.9429) centre (-27.681, 21.3193) ccw
  line L72 (-27.3516, 22.9429) -> (-28.4826, 22.9429)
  arc A83 (-30.5154, 20.1813) -> (-28.8838, 21.7204) centre (-30.366, 21.6573) ccw
  line L73 (-31.75, 23.2566) -> (-31.75, 22.8376)
  arc A84 (-30.7471, 25.8454) -> (-32.855, 25.8454) centre (-31.8011, 17.6506) ccw
  arc A85 (-28.8899, 24.3267) -> (-29.419, 25.3656) centre (-30.1804, 24.3237) ccw
  line L74 (-28.8838, 21.7204) -> (-28.8899, 24.3267)
  arc A86 (-32.855, 25.8454) -> (-34.2085, 25.3656) centre (-32.5939, 22.9597) ccw
  line L75 (-34.6167, 23.2566) -> (-31.75, 23.2566)
  arc A87 (-34.2085, 25.3656) -> (-34.6167, 24.7252) centre (-33.7105, 24.5979) ccw
  line L76 (-33.5029, 20.1743) -> (-30.5154, 20.1813)
  line L77 (-31.75, 22.8376) -> (-35.7944, 22.8376)
  arc A88 (-34.7452, 19.4922) -> (-35.005, 18.5598) centre (-33.1209, 18.5371) ccw
  arc A89 (-33.5029, 20.1743) -> (-34.7452, 19.4922) centre (-33.4773, 18.6554) ccw
  arc A90 (-29.419, 25.3656) -> (-30.7471, 25.8454) centre (-31.1247, 22.7218) ccw
  line L78 (-34.6167, 24.7252) -> (-34.6167, 23.2566)
  line L79 (-35.005, 17.0858) -> (-35.005, 18.5598)
  arc A91 (-35.7944, 22.8376) -> (-37.5375, 21.3277) centre (-35.7099, 20.979) ccw
  arc A92 (-37.345, 18.0946) -> (-36.136, 17.0858) centre (-35.8066, 18.7095) ccw
  arc A93 (-37.5375, 21.3277) -> (-37.345, 18.0946) centre (-32.5755, 20.0009) ccw
  line L80 (-36.136, 17.0858) -> (-35.005, 17.0858)
  circle A94 centre (-30.1167, 15.5587) radius 0.5161
  circle A95 centre (-33.3836, 24.5305) radius 0.545
  line L81 (-56.2312, 66.6599) -> (-56.2312, 67.7801)
  arc A96 (-56.0337, 68.4887) -> (-56.2312, 67.7801) centre (-54.7992, 67.7629) ccw
  arc A97 (-55.0896, 69.0071) -> (-56.0337, 68.4887) centre (-55.0701, 67.8527) ccw
  line L82 (-55.0896, 69.0071) -> (-52.8191, 69.0124)
  arc A98 (-52.8191, 69.0124) -> (-51.579, 70.1822) centre (-52.7055, 70.1342) ccw
  line L83 (-51.579, 70.1822) -> (-51.5837, 72.1629)
  arc A99 (-51.5837, 72.1629) -> (-51.9858, 72.9525) centre (-52.5644, 72.1606) ccw
  arc A100 (-51.9858, 72.9525) -> (-52.9952, 73.3171) centre (-53.2822, 70.9432) ccw
  arc A101 (-52.9952, 73.3171) -> (-54.5972, 73.3171) centre (-53.7962, 67.0891) ccw
  arc A102 (-54.5972, 73.3171) -> (-55.6258, 72.9525) centre (-54.3987, 71.124) ccw
  arc A103 (-55.6258, 72.9525) -> (-55.936, 72.4658) centre (-55.2474, 72.369) ccw
  line L84 (-55.936, 72.4658) -> (-55.936, 71.3496)
  line L85 (-55.936, 71.3496) -> (-53.7574, 71.3496)
  line L86 (-53.7574, 71.3496) -> (-53.7574, 71.0312)
  line L87 (-53.7574, 71.0312) -> (-56.8311, 71.0312)
  arc A104 (-56.8311, 71.0312) -> (-58.1558, 69.8837) centre (-56.7669, 69.6187) ccw
  arc A105 (-58.1558, 69.8837) -> (-58.0095, 67.4265) centre (-54.3847, 68.8753) ccw
  arc A106 (-58.0095, 67.4265) -> (-57.0907, 66.6599) centre (-56.8404, 67.8938) ccw
  line L88 (-57.0907, 66.6599) -> (-56.2312, 66.6599)
  arc A107 (-54.6862, 68.7587) -> (-55.9262, 67.5889) centre (-54.7998, 67.6369) ccw
  line L89 (-53.7479, 66.4215) -> (-53.7479, 66.7399)
  arc A108 (-54.5101, 64.454) -> (-52.9081, 64.454) centre (-53.7091, 70.682) ccw
  arc A109 (-55.9216, 65.6082) -> (-55.5195, 64.8186) centre (-54.9409, 65.6105) ccw
  line L90 (-55.9262, 67.5889) -> (-55.9216, 65.6082)
  arc A110 (-52.9081, 64.454) -> (-51.8795, 64.8186) centre (-53.1066, 66.6471) ccw
  line L91 (-51.5693, 66.4215) -> (-53.7479, 66.4215)
  arc A111 (-51.8795, 64.8186) -> (-51.5693, 65.3053) centre (-52.2579, 65.4021) ccw
  line L92 (-52.4157, 68.764) -> (-54.6862, 68.7587)
  line L93 (-53.7479, 66.7399) -> (-50.6742, 66.7399)
  arc A112 (-51.4716, 69.2824) -> (-51.2741, 69.991) centre (-52.7061, 70.0082) ccw
  arc A113 (-52.4157, 68.764) -> (-51.4716, 69.2824) centre (-52.4352, 69.9184) ccw
  arc A114 (-55.5195, 64.8186) -> (-54.5101, 64.454) centre (-54.2231, 66.8279) ccw
  line L94 (-51.5693, 65.3053) -> (-51.5693, 66.4215)
  line L95 (-51.2741, 71.1112) -> (-51.2741, 69.991)
  arc A115 (-50.6742, 66.7399) -> (-49.3495, 67.8874) centre (-50.7384, 68.1524) ccw
  arc A116 (-49.4958, 70.3446) -> (-50.4146, 71.1112) centre (-50.6649, 69.8773) ccw
  arc A117 (-49.3495, 67.8874) -> (-49.4958, 70.3446) centre (-53.1206, 68.8958) ccw
  line L96 (-50.4146, 71.1112) -> (-51.2741, 71.1112)
  circle A118 centre (-54.9893, 72.2719) radius 0.3922
  circle A119 centre (-52.5064, 65.4533) radius 0.4142
  line L97 (-12.2353, 17.7683) -> (-12.2353, 18.8885)
  arc A120 (-12.0378, 19.5971) -> (-12.2353, 18.8885) centre (-10.8033, 18.8713) ccw
  arc A121 (-11.0937, 20.1155) -> (-12.0378, 19.5971) centre (-11.0742, 18.9611) ccw
  line L98 (-11.0937, 20.1155) -> (-8.8232, 20.1208)
  arc A122 (-8.8232, 20.1208) -> (-7.5832, 21.2905) centre (-8.7096, 21.2425) ccw
  line L99 (-7.5832, 21.2905) -> (-7.5878, 23.2713)
  arc A123 (-7.5878, 23.2713) -> (-7.9899, 24.0609) centre (-8.5686, 23.269) ccw
  arc A124 (-7.9899, 24.0609) -> (-8.9993, 24.4255) centre (-9.2863, 22.0516) ccw
  arc A125 (-8.9993, 24.4255) -> (-10.6013, 24.4255) centre (-9.8003, 18.1974) ccw
  arc A126 (-10.6013, 24.4255) -> (-11.6299, 24.0609) centre (-10.4028, 22.2324) ccw
  arc A127 (-11.6299, 24.0609) -> (-11.9402, 23.5742) centre (-11.2515, 23.4774) ccw
  line L100 (-11.9402, 23.5742) -> (-11.9402, 22.458)
  line L101 (-11.9402, 22.458) -> (-9.7615, 22.458)
  line L102 (-9.7615, 22.458) -> (-9.7615, 22.1396)
  line L103 (-9.7615, 22.1396) -> (-12.8352, 22.1396)
  arc A128 (-12.8352, 22.1396) -> (-14.16, 20.992) centre (-12.771, 20.7271) ccw
  arc A129 (-14.16, 20.992) -> (-14.0136, 18.5349) centre (-10.3888, 19.9837) ccw
  arc A130 (-14.0136, 18.5349) -> (-13.0948, 17.7683) centre (-12.8445, 19.0022) ccw
  line L104 (-13.0948, 17.7683) -> (-12.2353, 17.7683)
  arc A131 (-10.6903, 19.8671) -> (-11.9304, 18.6973) centre (-10.8039, 18.7453) ccw
  line L105 (-9.7521, 17.5299) -> (-9.7521, 17.8482)
  arc A132 (-10.5142, 15.5624) -> (-8.9122, 15.5624) centre (-9.7132, 21.7904) ccw
  arc A133 (-11.9257, 16.7166) -> (-11.5236, 15.927) centre (-10.945, 16.7189) ccw
  line L106 (-11.9304, 18.6973) -> (-11.9257, 16.7166)
  arc A134 (-8.9122, 15.5624) -> (-7.8836, 15.927) centre (-9.1107, 17.7555) ccw
  line L107 (-7.5734, 17.5299) -> (-9.7521, 17.5299)
  arc A135 (-7.8836, 15.927) -> (-7.5734, 16.4137) centre (-8.2621, 16.5104) ccw
  line L108 (-8.4198, 19.8724) -> (-10.6903, 19.8671)
  line L109 (-9.7521, 17.8482) -> (-6.6783, 17.8482)
  arc A136 (-7.4757, 20.3908) -> (-7.2782, 21.0994) centre (-8.7102, 21.1166) ccw
  arc A137 (-8.4198, 19.8724) -> (-7.4757, 20.3908) centre (-8.4393, 21.0268) ccw
  arc A138 (-11.5236, 15.927) -> (-10.5142, 15.5624) centre (-10.2273, 17.9363) ccw
  line L110 (-7.5734, 16.4137) -> (-7.5734, 17.5299)